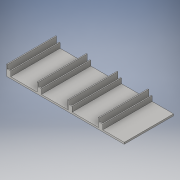
# Autodesk Inventor part: NewModuleHolder
Saved by Autodesk Inventor 2016 (Build 200138000, 138)
## iProperties
Created: 2016-11-23
Part Number: NewModuleHolder
Material: Generic
Document SubType Name: Modeling
Designer: RoboticsUser
Density: 1 g/cm^3
Appearance: Default
Author: RoboticsUser
Autodesk Inventor part; units mm, degrees
ref_plane "YZ Plane" through (0, 0, 0) normal (1, 0, 0) x (0, 1, 0)
ref_plane "XZ Plane" through (0, 0, 0) normal (0, 1, 0) x (-1, 0, 0)
ref_plane "XY Plane" through (0, 0, 0) normal (0, 0, 1) x (1, 0, 0)
sketch "Sketch1" plane through (0, 0, 0) normal (0, 0, 1) x (1, 0, 0)
  line L0 (0, 0) -> (206.4004, 0)
  line L1 (206.4004, 0) -> (206.4004, 2.9922)
  line L2 (206.4004, 2.9922) -> (0, 2.9922)
  line L3 (0, 2.9922) -> (0, 0)
  dimension "d0" = 206.4004
  constraints: 8 end point, 2 parallel, 1 horizontal, 1 perpendicular
  measures "d0" distance of L2.end L1.end
extrude "Extrusion1" add sketch "Sketch1" along normal blind 86.36
sketch "Sketch2" plane through (0, 2.9922, 0) normal (0, 1, 0) x (1, 0, 0)
  line L0 (0, -86.36) -> (206.4004, -86.36) projected
  line L1 (0, 0) -> (1.6002, 0)
  line L2 (1.6002, 0) -> (1.6002, -86.36)
  line L3 (1.6002, -86.36) -> (0, -86.36)
  line L4 (0, -86.36) -> (0, 0)
  dimension "d3" = 1.6002
  constraints: 8 end point, 2 parallel, 1 horizontal, 1 perpendicular, 1 point on line
  measures "d3" distance of L2.end L3.end
extrude "Extrusion2" add sketch "Sketch2" along normal blind 15.24
sketch "Sketch3" plane through (206.4004, 2.9922, 86.36) normal (0, 1, 0) x (1, 0, 0)
  line L0 (-206.4004, 86.36) -> (0, 86.36) projected
  line L1 (-200.4568, 0) -> (-198.8566, 0)
  line L2 (-198.8566, 0) -> (-198.8566, 86.36)
  line L3 (-198.8566, 86.36) -> (-200.4568, 86.36)
  line L4 (-200.4568, 86.36) -> (-200.4568, 0)
  dimension "d6" = 1.6002
  constraints: 8 end point, 2 parallel, 1 horizontal, 1 perpendicular, 1 point on line
  measures "d6" distance of L3.end L2.end
extrude "Extrusion3" add sketch "Sketch3" along normal blind 8.636
sketch "Sketch4" plane through (206.4004, 2.9922, 86.36) normal (0, 1, 0) x (1, 0, 0)
  line L0 (-206.4004, 86.36) -> (0, 86.36) projected
  line L1 (-152.654, 0) -> (-151.0538, 0)
  line L2 (-151.0538, 0) -> (-151.0538, 86.36)
  line L3 (-151.0538, 86.36) -> (-152.654, 86.36)
  line L4 (-152.654, 86.36) -> (-152.654, 0)
  dimension "d9" = 1.6002
  constraints: 8 end point, 2 parallel, 1 horizontal, 1 perpendicular, 1 point on line
  measures "d9" distance of L3.end L2.end
extrude "Extrusion4" add sketch "Sketch4" along normal blind 15.24
sketch "Sketch5" plane through (206.4004, 2.9922, 86.36) normal (0, 1, 0) x (1, 0, 0)
  line L0 (0, 0) -> (-151.0538, 0) projected
  line L1 (0, 86.36) -> (-151.0538, 86.36) projected
  line L2 (-146.7104, 0) -> (-145.1102, 0)
  line L3 (-145.1102, 0) -> (-145.1102, 86.36)
  line L4 (-145.1102, 86.36) -> (-146.7104, 86.36)
  line L5 (-146.7104, 86.36) -> (-146.7104, 0)
  point P0 (-206.4004, 86.36)
  dimension "d12" = 1.6002
  constraints: 8 end point, 2 parallel, 2 point on line, 1 horizontal, 1 perpendicular
  measures "d12" distance of L4.end L3.end
extrude "Extrusion5" add sketch "Sketch5" along normal blind 8.636
sketch "Sketch6" plane through (206.4004, 2.9922, 86.36) normal (0, 1, 0) x (1, 0, 0)
  line L0 (0, 86.36) -> (-145.1102, 86.36) projected
  line L1 (-98.9584, 0) -> (-97.3582, 0)
  line L2 (-97.3582, 0) -> (-97.3582, 86.36)
  line L3 (-97.3582, 86.36) -> (-98.9584, 86.36)
  line L4 (-98.9584, 86.36) -> (-98.9584, 0)
  point P0 (-206.4004, 86.36)
  dimension "d15" = 1.6002
  constraints: 8 end point, 2 parallel, 1 horizontal, 1 perpendicular, 1 point on line
  measures "d15" distance of L3.end L2.end
extrude "Extrusion6" add sketch "Sketch6" along normal blind 15.24
sketch "Sketch7" plane through (206.4004, 2.9922, 86.36) normal (0, 1, 0) x (1, 0, 0)
  line L0 (0, 86.36) -> (-97.3582, 86.36) projected
  line L1 (-93.0148, 0) -> (-91.4146, 0)
  line L2 (-91.4146, 0) -> (-91.4146, 86.36)
  line L3 (-91.4146, 86.36) -> (-93.0148, 86.36)
  line L4 (-93.0148, 86.36) -> (-93.0148, 0)
  point P0 (-206.4004, 86.36)
  dimension "d18" = 1.6002
  constraints: 8 end point, 2 parallel, 1 horizontal, 1 perpendicular, 1 point on line
  measures "d18" distance of L3.end L2.end
extrude "Extrusion7" add sketch "Sketch7" along normal blind 8.636
sketch "Sketch8" plane through (206.4004, 2.9922, 86.36) normal (0, 1, 0) x (1, 0, 0)
  line L0 (-206.4004, 0) -> (0, 0) projected
  line L1 (-206.4004, 86.36) -> (0, 86.36) projected
  line L2 (-45.212, 0) -> (-43.6118, 0)
  line L3 (-43.6118, 0) -> (-43.6118, 86.36)
  line L4 (-43.6118, 86.36) -> (-45.212, 86.36)
  line L5 (-45.212, 86.36) -> (-45.212, 0)
  dimension "d21" = 1.6002
  constraints: 8 end point, 2 parallel, 2 point on line, 1 horizontal, 1 perpendicular
  measures "d21" distance of L4.end L3.end
extrude "Extrusion8" add sketch "Sketch8" along normal blind 15.24
sketch "Sketch9" plane through (206.4004, 2.9922, 86.36) normal (0, 1, 0) x (1, 0, 0)
  line L0 (-206.4004, 0) -> (0, 0) projected
  line L1 (-206.4004, 86.36) -> (0, 86.36) projected
  line L2 (-39.2684, 0) -> (-37.6682, 0)
  line L3 (-37.6682, 0) -> (-37.6682, 86.36)
  line L4 (-37.6682, 86.36) -> (-39.2684, 86.36)
  line L5 (-39.2684, 86.36) -> (-39.2684, 0)
  dimension "d24" = 1.6002
  constraints: 8 end point, 2 parallel, 2 point on line, 1 horizontal, 1 perpendicular
  measures "d24" distance of L4.end L3.end
extrude "Extrusion9" add sketch "Sketch9" along normal blind 8.636
sketch "Sketch10" plane through (109.0422, 2.9922, 86.36) normal (0, 1, 0) x (1, 0, 0)
  line L0 (-109.0422, 0) -> (97.3582, 0) projected
  line L1 (4.3434, 86.36) -> (4.3434, 0) projected
  line L2 (0.0002, 0) -> (4.3434, 0)
  line L3 (4.3434, 0) -> (4.3434, 1.6002)
  line L4 (4.3434, 1.6002) -> (0.0002, 1.6002)
  line L5 (0.0002, 1.6002) -> (0.0002, 0)
  point P0 (-109.0422, 86.36)
  dimension "d27" = 1.6002
  constraints: 8 end point, 2 parallel, 2 point on line, 1 horizontal, 1 perpendicular
  measures "d27" distance of L3.end L2.end
extrude "Extrusion10" add sketch "Sketch10" along normal blind 8.636
sketch "Sketch11" plane through (162.7886, 2.9922, 86.36) normal (0, 1, 0) x (1, 0, 0)
  line L0 (0, 0) -> (0, 86.36) projected
  line L1 (4.3434, 86.36) -> (4.3434, 0) projected
  line L2 (0, 0) -> (4.3434, 0)
  line L3 (4.3434, 0) -> (4.3434, 1.5956)
  line L4 (4.3434, 1.5956) -> (0, 1.5956)
  line L5 (0, 1.5956) -> (0, 0)
  point P0 (-162.7886, 86.36)
  constraints: 8 end point, 2 parallel, 1 horizontal, 1 perpendicular, 1 point on line
extrude "Extrusion11" add sketch "Sketch11" along normal blind 8.636
sketch "Sketch12" plane through (55.3466, 2.9922, 86.36) normal (0, 1, 0) x (1, 0, 0)
  line L0 (4.3434, 0) -> (0, 0) projected
  line L1 (4.3434, 86.36) -> (4.3434, 0) projected
  line L2 (0, 0) -> (4.3434, 0)
  line L3 (4.3434, 0) -> (4.3434, 1.5937)
  line L4 (4.3434, 1.5937) -> (0, 1.5937)
  line L5 (0, 1.5937) -> (0, 0)
  point P0 (-55.3466, 86.36)
  constraints: 8 end point, 2 parallel, 1 horizontal, 1 perpendicular, 1 point on line
extrude "Extrusion12" add sketch "Sketch12" along normal blind 8.636
sketch "Sketch13" plane through (1.6002, 2.9922, 86.36) normal (0, 1, 0) x (1, 0, 0)
  line L0 (4.3434, 86.36) -> (4.3434, 0) projected
  line L1 (0, 0) -> (4.3434, 0)
  line L2 (4.3434, 0) -> (4.3434, 1.6077)
  line L3 (4.3434, 1.6077) -> (0, 1.6077)
  line L4 (0, 1.6077) -> (0, 0)
  point P0 (-1.6002, 86.36)
  constraints: 8 end point, 2 parallel, 1 horizontal, 1 perpendicular, 1 point on line
extrude "Extrusion13" add sketch "Sketch13" along normal blind 8.636
body "Solid1"
